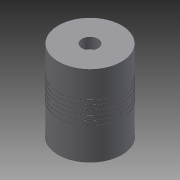
# Autodesk Inventor part: Shaft_Coupler_5mm_10mm
Saved by Autodesk Inventor 2015 (Build 190159000, 159)
## iProperties
Created: 2014-12-22
Part Number: Shaft_Coupler_5mm_10mm
Material: Generic
Document SubType Name: Modeling
Designer: Drew
Density: 1 g/cm^3
Appearance: Default
Author: Drew
Autodesk Inventor part; units mm, degrees
ref_plane "YZ Plane" through (0, 0, 0) normal (1, 0, 0) x (0, 1, 0)
ref_plane "XZ Plane" through (0, 0, 0) normal (0, 1, 0) x (-1, 0, 0)
ref_plane "XY Plane" through (0, 0, 0) normal (0, 0, 1) x (1, 0, 0)
sketch "Sketch2" plane through (0, 0, 0) normal (1, 0, 0) x (0, 1, 0)
  line L0 (3.3337, 0) -> (3.3337, -5)
  line L1 (3.3337, -5) -> (0, -5)
  line L2 (0, -5) -> (0, -10)
  line L3 (25.4, -10) -> (25.4, -2.5)
  line L4 (25.4, -2.5) -> (22.2077, -2.5)
  line L5 (22.2077, -2.5) -> (22.2077, 0)
  line L6 (17.1277, 0) -> (17.1277, -10)
  line L7 (17.0007, -10) -> (17.0007, 0)
  line L8 (22.2077, 0) -> (17.1277, 0)
  line L9 (17.1277, -10) -> (25.4, -10)
  line L10 (15.7307, 0) -> (15.7307, -10)
  line L11 (15.6037, 0) -> (15.6037, -10)
  line L12 (14.3337, 0) -> (14.3337, -10)
  line L13 (14.2067, 0) -> (14.2067, -10)
  line L14 (15.7307, -10) -> (17.0007, -10)
  line L15 (17.0007, 0) -> (15.7307, 0)
  line L16 (15.6037, 0) -> (14.3337, 0)
  line L17 (14.3337, -10) -> (15.6037, -10)
  line L18 (12.9367, 0) -> (12.9367, -10)
  line L19 (12.8097, -10) -> (12.8097, 0)
  line L20 (11.5397, 0) -> (11.5397, -10)
  line L21 (11.4127, -10) -> (11.4127, 0)
  line L22 (10.1427, 0) -> (10.1427, -10)
  line L23 (10.0157, -10) -> (10.0157, 0)
  line L24 (14.2067, 0) -> (12.9367, 0)
  line L25 (12.9367, -10) -> (14.2067, -10)
  line L26 (11.5397, -10) -> (12.8097, -10)
  line L27 (12.8097, 0) -> (11.5397, 0)
  line L28 (11.4127, 0) -> (10.1427, 0)
  line L29 (10.0157, 0) -> (3.3337, 0)
  line L30 (0, -10) -> (10.0157, -10)
  line L31 (10.1427, -10) -> (11.4127, -10)
  point P0 (0, 0)
  dimension "d1" = 3.1923
  dimension "d2" = 3.3337
  dimension "d3" = 25.4
  dimension "d4" = 0.127
  dimension "d5" = 0.127
  dimension "d6" = 0.127
  dimension "d7" = 0.127
  dimension "d8" = 0.127
  dimension "d10" = 0.127
  dimension "d12" = 1.27
  dimension "d13" = 1.27
  dimension "d14" = 1.27
  dimension "d15" = 1.27
  dimension "d16" = 1.27
  dimension "d17" = 2.5
  dimension "d18" = 5
  dimension "d20" = 10
  dimension "d21" = 5.08
  constraints: 86 perpendicular, 64 end point, 7 horizontal, 6 collinear, 2 vertical
  measures "d1" distance of L3.end L4.end
  measures "d2" distance of L0.end L1.end
  measures "d3" distance between parallel lines of L3 L2
  measures "d4" distance between parallel lines of L6 L7
  measures "d5" distance between parallel lines of L11 L10
  measures "d6" distance between parallel lines of L12 L13
  measures "d7" distance between parallel lines of L18 L19
  measures "d8" distance between parallel lines of L20 L21
  measures "d10" distance between parallel lines of L22 L23
  measures "d12" distance between parallel lines of L11 L12
  measures "d13" distance between parallel lines of L13 L18
  measures "d14" distance between parallel lines of L19 L20
  measures "d15" distance between parallel lines of L21 L22
  measures "d16" distance between parallel lines of L7 L10
  measures "d17" distance of L4.end L5.end
  measures "d18" distance of L0.start L0.end
  measures "d20" distance between parallel lines of L8 L9
  measures "d21" distance between parallel lines of L5 L6
revolve "Revolution2" add sketch "Sketch2" angle 360 about axis through (0, 22.2077, 0) along (0, -1, 0)
equation "\"d5\" = d4"
equation "\"d6\" = d5"
equation "\"d7\" = d6"
equation "\"d8\" = d7"
equation "\"d10\" = d8"
equation "\"d13\" = d12"
equation "\"d14\" = d13"
equation "\"d15\" = d14"
equation "\"d16\" = d12"
body "Solid2"
